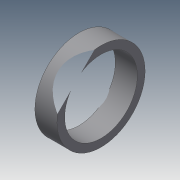
# Autodesk Inventor part: Wheel
Saved by Autodesk Inventor 2014 SP1 (Build 180222100, 222)
## iProperties
Created: 2014-01-20
Part Number: Wheel
Material: Generic
Document SubType Name: Modeling
Designer: tom
Density: 1 g/cm^3
Appearance: Default
d0: 4.000 in
d1: 0.500 in
d2: 0.770 in
d3: 1.500 in
d4: 2.000 in
d5: 2.500 in
d6: 3.000 in
d7: 3.300 in
d17: 0.250 in
d18: 0.00 deg
d19: 4.000 in
d20: 0.500 in
d21: 0.770 in
d22: 1.500 in
d23: 2.000 in
d24: 2.500 in
d25: 3.000 in
d26: 3.300 in
d27: 0.140 in
d28: 0.140 in
d29: 0.140 in
d30: 0.140 in
d31: 0.140 in
d32: 1.000 in
d33: 0.00 deg
d34: 4.000 in
d35: 0.500 in
d36: 0.770 in
d37: 1.500 in
d38: 2.000 in
d39: 2.500 in
d40: 3.000 in
d41: 3.300 in
d42: 0.140 in
d43: 0.140 in
d44: 0.140 in
d45: 0.140 in
d46: 0.140 in
d47: 0.250 in
d48: 0.00 deg
d49: 8.000 ul
d50: 360.00 deg
d53: 0.063 in
d54: 0.250 in
d55: 0.00 deg
d56: 8.000 ul
d57: 360.00 deg
Author: tom
Autodesk Inventor part; units mm, degrees
ref_plane "YZ Plane" through (0, 0, 0) normal (1, 0, 0) x (0, 1, 0)
ref_plane "XZ Plane" through (0, 0, 0) normal (0, 1, 0) x (-1, 0, 0)
ref_plane "XY Plane" through (0, 0, 0) normal (0, 0, 1) x (1, 0, 0)
sketch "Sketch1" plane through (0, 0, 0) normal (1, 0, 0) x (0, 1, 0)
  circle A0 centre (0, 0) radius 50.8
  circle A1 centre (0, 0) radius 6.35
  circle A2 centre (0, 0) radius 9.779 construction
  circle A3 centre (0, 0) radius 19.05 construction
  circle A4 centre (0, 0) radius 25.4 construction
  circle A5 centre (0, 0) radius 31.75 construction
  circle A6 centre (0, 0) radius 38.1 construction
  circle A7 centre (0, 0) radius 41.91
  line L0 (0, 0) -> (41.91, 0) construction
  line L1 (0, 50.8) -> (0, -50.8) construction
  dimension "d0" = 101.6
  dimension "d1" = 12.7
  dimension "d2" = 19.558
  dimension "d3" = 38.1
  dimension "d4" = 50.8
  dimension "d5" = 63.5
  dimension "d6" = 76.2
  dimension "d7" = 83.82
  constraints: 8 centre point, 8 coincident, 4 end point, 2 point on circle, 1 horizontal, 1 perpendicular
  measures "d0" diameter of A0
  measures "d1" diameter of A1
  measures "d2" diameter of A2
  measures "d3" diameter of A3
  measures "d4" diameter of A4
  measures "d5" diameter of A5
  measures "d6" diameter of A6
  measures "d7" diameter of A7
extrude "Extrusion1" add sketch "Sketch1" along normal mid plane 6.35 contours A7
sketch "Sketch2" plane through (0, 0, 0) normal (1, 0, 0) x (0, 1, 0)
  circle A0 centre (0, 0) radius 50.8
  circle A1 centre (0, 0) radius 6.35
  circle A2 centre (0, 0) radius 9.779 construction
  circle A3 centre (0, 0) radius 19.05 construction
  circle A4 centre (0, 0) radius 25.4 construction
  circle A5 centre (0, 0) radius 31.75 construction
  circle A6 centre (0, 0) radius 38.1 construction
  circle A7 centre (0, 0) radius 41.91
  line L0 (0, 0) -> (41.91, 0) construction
  line L1 (0, 50.8) -> (0, -50.8) construction
  circle A8 centre (0, 9.779) radius 1.778
  circle A9 centre (0, 19.05) radius 1.778
  circle A10 centre (0, 25.4) radius 1.778
  circle A11 centre (0, 31.75) radius 1.778
  circle A12 centre (0, 38.1) radius 1.778
  dimension "d21" = 19.558
  dimension "d22" = 38.1
  dimension "d23" = 50.8
  dimension "d24" = 63.5
  dimension "d25" = 76.2
  dimension "d19" = 101.6
  dimension "d20" = 12.7
  dimension "d26" = 83.82
  dimension "d27" = 3.556
  dimension "d28" = 3.556
  dimension "d29" = 3.556
  dimension "d30" = 3.556
  dimension "d31" = 3.556
  constraints: 8 centre point, 8 coincident, 5 vertical alignment, 4 end point, 4 point on line, 2 point on circle, 1 horizontal, 1 perpendicular, 10 other
  measures "d19" diameter of A0
  measures "d20" diameter of A1
  measures "d26" diameter of A7
  measures "d27" diameter of A8
  measures "d28" diameter of A9
  measures "d29" diameter of A10
  measures "d30" diameter of A11
  measures "d31" diameter of A12
extrude "Extrusion2" add sketch "Sketch2" along normal mid plane 25.4 contours A0
sketch "Sketch4" plane through (3.175, 0, 0) normal (1, 0, 0) x (0, 0, -1)
  circle A0 centre (0, 0) radius 50.8
  circle A1 centre (0, 0) radius 6.35
  circle A2 centre (0, 0) radius 9.779 construction
  circle A3 centre (0, 0) radius 19.05 construction
  circle A4 centre (0, 0) radius 25.4 construction
  circle A5 centre (0, 0) radius 31.75 construction
  circle A6 centre (0, 0) radius 38.1 construction
  circle A7 centre (0, 0) radius 41.91
  line L0 (0, 0) -> (41.91, 0) construction
  line L1 (0, 50.8) -> (0, -50.8) construction
  circle A8 centre (0, 9.779) radius 1.778
  circle A9 centre (0, 19.05) radius 1.778
  circle A10 centre (0, 25.4) radius 1.778
  circle A11 centre (0, 31.75) radius 1.778
  circle A12 centre (0, 38.1) radius 1.778
  dimension "d36" = 19.558
  dimension "d37" = 38.1
  dimension "d38" = 50.8
  dimension "d39" = 63.5
  dimension "d40" = 76.2
  dimension "d34" = 101.6
  dimension "d35" = 12.7
  dimension "d41" = 83.82
  dimension "d42" = 3.556
  dimension "d43" = 3.556
  dimension "d44" = 3.556
  dimension "d45" = 3.556
  dimension "d46" = 3.556
  constraints: 8 centre point, 8 coincident, 5 vertical alignment, 4 end point, 4 point on line, 2 point on circle, 1 horizontal, 1 perpendicular, 10 other
  measures "d34" diameter of A0
  measures "d35" diameter of A1
  measures "d41" diameter of A7
  measures "d42" diameter of A8
  measures "d43" diameter of A9
  measures "d44" diameter of A10
  measures "d45" diameter of A11
  measures "d46" diameter of A12
extrude "Extrusion3" cut sketch "Sketch4" against normal blind 6.35 contours A8 | A9 | A10 | A11 | A12
pattern_circular "Circular Pattern1" count 8 over 360 about axis through (0, 0, 0) along (1, 0, 0) of "Extrusion3"
sketch "Sketch5" plane through (3.175, 0, 0) normal (1, 0, 0) x (0, 0, -1)
  circle A0 centre (38.1, 0) radius 1.778 projected
  circle A1 centre (6.9148, -6.9148) radius 1.778 projected
  circle A2 centre (-6.9148, 6.9148) radius 1.778 projected
  circle A3 centre (0, 0) radius 6.35 projected
  circle A4 centre (0, 0) radius 41.91 projected
  line L0 (-6.35, 0) -> (-6.35, 39.3692) construction
  line L1 (6.35, 19.1628) -> (6.35, 37.4588) construction
  line L2 (-6.9148, 6.9148) -> (6.9148, -6.9148) construction
  line L3 (4.4901, -4.4901) -> (32.3283, 23.3481) construction
  line L4 (9.06, 18.0403) -> (21.9972, 30.9775) construction
  line L5 (6.35, 19.1628) -> (6.35, 37.4588)
  line L6 (9.06, 18.0403) -> (21.9972, 30.9775)
  arc A5 (21.7401, 33.4308) -> (8.2666, 39.0118) centre (0, 0) ccw
  arc A6 (23.3481, 32.3283) -> (8.2666, 39.0118) centre (0, 0) ccw construction
  arc A7 (8.2666, 39.0118) -> (6.35, 37.4588) centre (7.9375, 37.4588) ccw
  arc A8 (6.35, 19.1628) -> (9.06, 18.0403) centre (7.9375, 19.1628) ccw
  arc A9 (21.9972, 30.9775) -> (21.7401, 33.4308) centre (20.8747, 32.1) ccw
  point P0 (6.35, 0)
  point P1 (-4.4901, 4.4901)
  point P2 (39.878, 0)
  dimension "d53" = 1.5875
  constraints: 15 point on circle, 14 end point, 10 tangent, 5 centre point, 5 point on line, 2 coincident, 2 collinear, 2 equal radius, 2 parallel, 1 horizontal alignment, 1 perpendicular, 1 vertical, 1 other
  measures "d53" radius of A7
extrude "Extrusion4" cut sketch "Sketch5" against normal blind 6.35 contours L5 A7 A5 A9 L6 A8
pattern_circular "Circular Pattern2" count 8 over 360 about axis through (0, 0, 0) along (1, 0, 0) of "Extrusion4"
body "Solid1"
